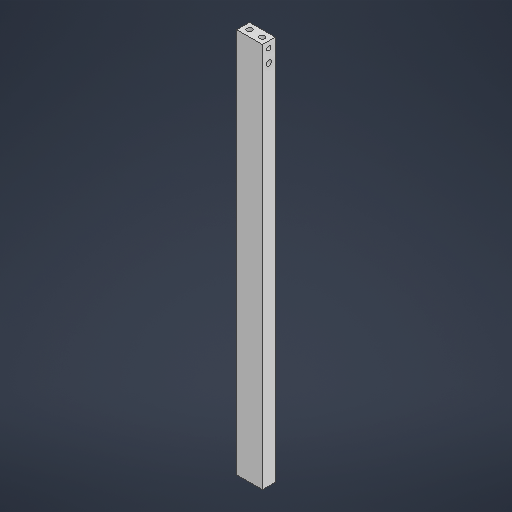
# Autodesk Inventor part: spine
Saved by Autodesk Inventor 2026 (Build 300175000, 175)
## iProperties
Created: 2025-07-17
Part Number: spine
Material: Generic
Document SubType Name: Modeling
Designer: User
Density: 1 g/cm^3
Appearance: Default
Author: User
Autodesk Inventor part; units mm, degrees
ref_plane "YZ Plane" through (0, 0, 0) normal (1, 0, 0) x (0, 1, 0)
ref_plane "XZ Plane" through (0, 0, 0) normal (0, 1, 0) x (-1, 0, 0)
ref_plane "XY Plane" through (0, 0, 0) normal (0, 0, 1) x (1, 0, 0)
sketch "Sketch1" plane through (0, 0, 0) normal (0, 1, 0) x (-1, 0, 0)
  line L0 (-10, 5) -> (10, 5)
  line L1 (10, 5) -> (10, -5)
  line L2 (10, -5) -> (-10, -5)
  line L3 (-10, -5) -> (-10, 5)
  line L4 (-10, 5) -> (10, -5) construction
  line L5 (10, 5) -> (-10, -5) construction
  point P0 (0, 0)
  dimension "d0" = 20
  dimension "d1" = 10
  constraints: 12 end point, 2 midpoint, 2 parallel, 1 horizontal, 1 perpendicular
  measures "d0" distance of L1.end L2.end
  measures "d1" distance of L0.end L1.end
extrude "Extrusion1" add sketch "Sketch1" along normal blind 300
sketch "Sketch2" plane through (0, 300, 0) normal (0, 1, 0) x (1, 0, 0)
  line L0 (0, 0) -> (0, 3.3139) construction
  line L1 (10, 5) -> (-10, 5) projected
  circle A0 centre (-5, 0) radius 2
  circle A1 centre (5, 0) radius 2
  line L2 (0, 0) -> (-5, 0)
  line L3 (0, 0) -> (5, 0)
  dimension "d4" = 4
  dimension "d7" = 5
  dimension "d8" = 5
  constraints: 6 end point, 2 centre point, 2 horizontal, 1 symmetric about line, 1 vertical, 1 other
  measures "d4" diameter of A0
  measures "d7" distance of L0.start L2.end
  measures "d8" distance of L0.start L3.end
extrude "Extrusion2" cut sketch "Sketch2" against normal blind 300
sketch "Sketch3" plane through (-10, 0, -5) normal (-1, 0, 0) x (0, 0, 1)
  line L0 (0, 300) -> (10, 300) projected
  line L1 (5, 300) -> (5, 295) construction
  line L2 (5, 295) -> (5, 285) construction
  circle A0 centre (5, 295) radius 1.6538
  circle A1 centre (5, 285) radius 2
  point P0 (5, 0)
  dimension "d9" = 5
  dimension "d10" = 10
  dimension "d11" = 4
  constraints: 4 end point, 2 centre point, 2 coincident, 1 midpoint, 1 point on line, 1 vertical
  measures "d9" distance of L1.start L1.end
  measures "d10" distance of L1.end L2.end
  measures "d11" diameter of A1
extrude "Extrusion3" cut sketch "Sketch3" against normal blind 32.225
body "Solid1"
